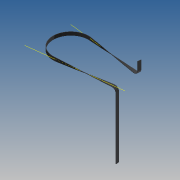
# Autodesk Inventor part: end belt
Saved by Autodesk Inventor 2013 (Build 170138000, 138)
## iProperties
Created: 2017-04-02
Part Number: end belt
Material: Generic
Document SubType Name: Modeling
Designer: employee
Density: 1 g/cm^3
Author: employee
Autodesk Inventor part; units mm, degrees
ref_plane "YZ Plane" through (0, 0, 0) normal (1, 0, 0) x (0, 1, 0)
ref_plane "XZ Plane" through (0, 0, 0) normal (0, 1, 0) x (-1, 0, 0)
ref_plane "XY Plane" through (0, 0, 0) normal (0, 0, 1) x (1, 0, 0)
sketch "Sketch1" plane through (0, 0, 0) normal (0, 0, 1) x (1, 0, 0)
  circle A0 centre (0, 0) radius 31.830989
  circle A1 centre (0, 0) radius 32.205989
  circle A2 centre (0, 0) radius 31.576989
  dimension "d0" = 63.66198
  dimension "d2" = 0.254
  dimension "d3" = 0.375
  constraints: 3 centre point, 1 coincident
  measures "d0" diameter of A0
  measures "d2" radial gap between concentric circles of A0 A2
  measures "d3" radial gap between concentric circles of A1 A0
sketch "Sketch1 outline for Extrusion1" plane through (0, 0, 0) normal (0, 0, 1) x (1, 0, 0)
  circle A0 centre (0, 0) radius 32.205989
  circle A1 centre (0, 0) radius 31.576989
extrude "Extrusion1" add sketch "Sketch1 outline for Extrusion1" along normal blind 6
sketch "Sketch2" plane through (0, 0, 6) normal (0, 0, 1) x (1, 0, 0)
  circle A0 centre (0, 0) radius 32.205989
  line L0 (0, 0) -> (3.816108, 31.979103)
  line L1 (0, 0) -> (3.816108, -31.979103)
  dimension "d6" = 166.39
  constraints: 4 end point, 2 point on circle, 1 vertical alignment
  measures "d6" angle of L0 L1
extrude "Extrusion2" cut sketch "Sketch2" against normal through all contours A0 L1 L0 picked at (21.157827, -2.572713)
sketch "Sketch3" plane through (3.816108, 31.979103, 6) normal (0.9929552, -0.1184906, 0) x (0, 0, -1)
  line L0 (6, 0) -> (6, -0.629) projected
  line L1 (0, 0) -> (6, 0) projected
  line L2 (0, -0.629) -> (0, 0) projected
  line L3 (6, -0.629) -> (0, -0.629) projected
  point P0 (6, -32.205989)
  point P1 (3, -0.375)
  point P2 (3, -0.629)
  dimension "d9" = 0.254
  constraints: 1 midpoint, 1 vertical alignment
  measures "d9" distance from line of point (3, -0.375) L3
coil "Coil1" sketch "Sketch3" operation add axis through (3.771674, 31.606745, 3) along (0.9929552, -0.1184906, 0) pitch 371.456 turns 0.25 hand right
sketch "Sketch4" plane through (3.741577, -31.354534, 6) normal (0.9929552, 0.1184906, 0) x (0, 0, -1)
  line L0 (6, 0) -> (6, -0.629) projected
  line L1 (0, 0) -> (6, 0) projected
  line L2 (0, -0.629) -> (0, 0) projected
  line L3 (6, -0.629) -> (0, -0.629) projected
  point P0 (6, 31.576989)
  point P1 (3, -0.254)
  point P2 (3, 0)
  dimension "d18" = 0.254
  constraints: 1 midpoint, 1 vertical alignment
  measures "d18" distance from line of L1 point (3, -0.254)
coil "Coil2" sketch "Sketch4" operation add axis through (3.771674, -31.606745, 3) along (0.9929552, 0.1184906, 0) pitch 371.456 turns 0.25 hand right
sketch "Sketch5" plane through (95.625991, -17.624366, 3.254) normal (0.9929552, 0.1184906, 0) x (0, 0, -1)
  line L0 (0.629, 0) -> (0.629, -6)
  line L1 (0, 0) -> (0.629, 0)
  line L2 (0, -6) -> (0, 0)
  line L3 (0.629, -6) -> (0, -6)
  line L4 (7.629, 3.824142) -> (7.629, -17.635602)
  point P0 (3.254, 28.830989)
  dimension "d27" = 7
  constraints: 2 end point, 1 perpendicular
  measures "d27" distance between parallel lines of L0 L4
revolve "Revolution1" add sketch "Sketch5" angle 90 about axis through (95.172866, -13.827165, -4.375) along (-0.1184906, 0.9929552, 0)
sketch "Sketch6" plane through (96.336935, 23.582097, 3.375) normal (0.9929552, -0.1184906, 0) x (0, 0, -1)
  line L0 (0.629, 0) -> (0.629, -6)
  line L1 (0, 0) -> (0.629, 0)
  line L2 (0, -6) -> (0, 0)
  line L3 (0.629, -6) -> (0, -6)
  line L4 (-7, 6.068729) -> (-7, -13.038094)
  point P0 (3.375, -34.830989)
  dimension "d29" = 7
  constraints: 2 end point, 1 perpendicular
  measures "d29" distance between parallel lines of L4 L2
revolve "Revolution2" add sketch "Sketch6" angle 90 about axis through (97.056022, 29.608074, 10.375) along (-0.1184906, -0.9929552, 0)
sketch "Sketch9" plane through (96.336935, -23.582097, 2.625) normal (0.1184906, -0.9929552, 0) x (0.9929552, 0.1184906, 0)
  line L0 (7, -7) -> (7.629, -7)
  line L1 (7.629, -7) -> (7.629, -96.263661)
  line L2 (7.629, -96.263661) -> (7, -96.263661)
  line L3 (7, -96.263661) -> (7, -7)
  line L4 (-19.311334, -96.263661) -> (32.837796, -96.263661)
  point P0 (-92.864, -2.625)
  constraints: 8 end point, 2 parallel, 1 horizontal, 1 perpendicular, 1 point on line
extrude "Extrusion5" add sketch "Sketch9" against normal up to surface (6 mm away)
sketch "Sketch8" plane through (96.336935, 23.582097, 3.375) normal (0.1184906, 0.9929552, 0) x (0.9929552, -0.1184906, 0)
  line L0 (7, -7) -> (7.629, -7)
  line L1 (7.629, -7) -> (7.629, -42.986339)
  line L2 (7.629, -42.986339) -> (7, -42.986339)
  line L3 (7, -42.986339) -> (7, -7)
  line L4 (-19.443403, -42.986339) -> (32.667261, -42.986339)
  point P0 (-92.864, 3.375)
  constraints: 8 end point, 2 parallel, 1 horizontal, 1 perpendicular, 1 point on line
extrude "Extrusion4" add sketch "Sketch8" against normal up to surface (6 mm away)
body "Solid1"
